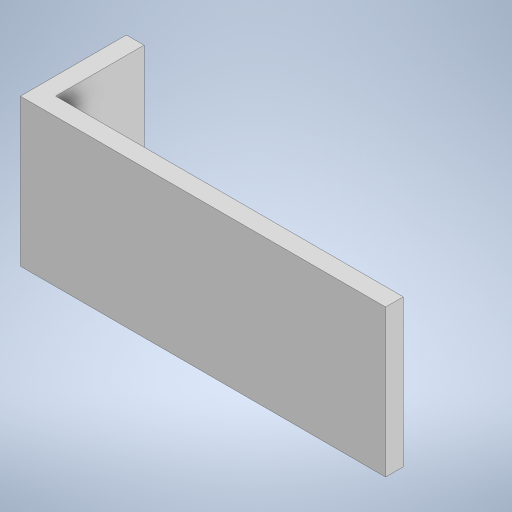
# Autodesk Inventor part: arduino array box v03 slot
Saved by Autodesk Inventor 2023 (Build 270158000, 158)
## iProperties
Created: 2024-07-14
Part Number: arduino array box v03 slot
Material: Generic
Document SubType Name: Modeling
Designer: Akramilab
Density: 1 g/cm^3
Appearance: Default
Author: Akramilab
Autodesk Inventor part; units mm, degrees
ref_plane "YZ Plane" through (0, 0, 0) normal (1, 0, 0) x (0, 1, 0)
ref_plane "XZ Plane" through (0, 0, 0) normal (0, 1, 0) x (-1, 0, 0)
ref_plane "XY Plane" through (0, 0, 0) normal (0, 0, 1) x (1, 0, 0)
sketch "Sketch1" plane through (0, 0, 0) normal (0, 0, 1) x (1, 0, 0)
  line L0 (0, 0) -> (59, 0)
  line L1 (59, 0) -> (59, -25)
  line L2 (59, -25) -> (0, -25)
  line L3 (0, -25) -> (0, 0)
  dimension "d0" = 59
  dimension "d1" = 25
  constraints: 8 end point, 2 parallel, 1 horizontal, 1 perpendicular
  measures "d0" distance of L1.end L2.end
  measures "d1" distance of L0.end L1.end
extrude "Extrusion1" add sketch "Sketch1" along normal blind 3
sketch "Sketch2" plane through (0, -25, 0) normal (-1, 0, 0) x (0, 0, 1)
  line L0 (3, 0) -> (3, 25) projected
  line L1 (3, 25) -> (-15, 25)
  line L2 (-15, 25) -> (-15, 0)
  line L3 (-15, 0) -> (3, 0)
  line L4 (3, 0) -> (3, 25)
  point P0 (0, 25)
  dimension "d4" = 18
  constraints: 8 end point, 2 parallel, 1 horizontal, 1 perpendicular
  measures "d4" distance of L3.end L2.end
extrude "Extrusion2" add sketch "Sketch2" along normal blind 3
body "Solid1"
